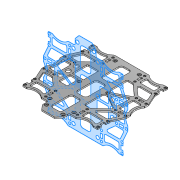
# Autodesk Inventor part: 16_039_BOTTOM_CHASSIS_R1
Saved by Autodesk Inventor 2021.2 (Build 252289000, 289)
## iProperties
Created: 2018-08-08
Part Number: 16_039_BOTTOM_CHASSIS_R1
Material: アルミニウム 6061
Document SubType Name: Modeling
Designer: student
Density: 2.7 g/cm^3
Appearance: 機械加工 - アルミニウム
Mass: 38.4013 g
Surface Area: 190.865 cm^2
Volume: 14.2227 cm^3
Author: student
Autodesk Inventor part; units mm, degrees
ref_plane "YZ Plane" through (0, 0, 0) normal (1, 0, 0) x (0, 1, 0)
ref_plane "XZ Plane" through (0, 0, 0) normal (0, 1, 0) x (-1, 0, 0)
ref_plane "XY Plane" through (0, 0, 0) normal (0, 0, 1) x (1, 0, 0)
sketch "スケッチ1" plane through (0, 0, 0) normal (0, 0, 1) x (1, 0, 0)
  arc A0 (80, 0) -> (40, 69.282) centre (0, 0) ccw construction
  line L0 (0, 0) -> (40, 69.282) construction
  line L1 (0, 0) -> (47.25, 0) construction
  circle A1 centre (24.25, 51.532) radius 1.05
  circle A2 centre (24.25, 36.532) radius 1.05
  circle A3 centre (55.75, 51.532) radius 1.05
  circle A4 centre (55.75, 36.532) radius 1.05
  line L2 (57.25, 54.032) -> (51.25, 54.032)
  line L3 (57.25, 54.032) -> (57.25, 52.8549)
  line L4 (57.25, 47.082) -> (55.2607, 47.082)
  line L5 (54.2, 47.082) -> (54.2, 46.0214) construction
  line L6 (54.2, 40.982) -> (55.2607, 40.982) construction
  line L7 (57.25, 40.982) -> (57.25, 37.8549)
  arc A5 (55.2607, 47.082) -> (54.2, 46.0214) centre (54.7303, 46.5517) ccw
  arc A6 (54.2, 42.0427) -> (55.2607, 40.982) centre (54.7303, 41.5124) ccw
  line L8 (55.2607, 47.082) -> (54.2, 47.082) construction
  line L9 (54.2, 46.0214) -> (54.2, 42.0427)
  line L10 (54.2, 42.0427) -> (54.2, 40.982) construction
  line L11 (55.2607, 40.982) -> (57.25, 40.982)
  line L12 (57.25, 34.032) -> (64.75, 17.25)
  line L13 (64.75, 17.25) -> (64.75, 11.25)
  arc A7 (27.0293, 55.7226) -> (50.6808, 53.8542) centre (40, 69.282) ccw
  arc A8 (64.5722, 10.6808) -> (64.5722, -10.6808) centre (80, 0) ccw
  arc A9 (51.25, 54.032) -> (50.6808, 53.8542) centre (51.25, 53.032) ccw
  arc A10 (27.0293, 55.7226) -> (26.3381, 56) centre (26.3381, 55) ccw
  line L14 (22.7, 40.982) -> (23.7607, 40.982) construction
  line L15 (25.8, 40.982) -> (25.8, 42.0427) construction
  line L16 (25.8, 47.082) -> (24.7393, 47.082) construction
  line L17 (22.7, 47.082) -> (22.7, 46.0214) construction
  arc A11 (22.7, 42.0427) -> (23.7607, 40.982) centre (23.2303, 41.5124) ccw
  arc A12 (23.7607, 47.082) -> (22.7, 46.0214) centre (23.2303, 46.5517) ccw
  arc A13 (25.8, 46.0214) -> (24.7393, 47.082) centre (25.2697, 46.5517) ccw
  arc A14 (24.7393, 40.982) -> (25.8, 42.0427) centre (25.2697, 41.5124) ccw
  line L18 (22.7, 46.0214) -> (22.7, 42.0427)
  line L19 (23.7607, 47.082) -> (22.7, 47.082) construction
  line L20 (24.7393, 47.082) -> (23.7607, 47.082)
  line L21 (25.8, 46.0214) -> (25.8, 47.082) construction
  line L22 (24.7393, 40.982) -> (25.8, 40.982) construction
  line L23 (25.8, 42.0427) -> (25.8, 46.0214)
  line L24 (23.7607, 40.982) -> (24.7393, 40.982)
  line L25 (22.7, 42.0427) -> (22.7, 40.982) construction
  line L26 (0, 56) -> (0, 0)
  arc A15 (64.5722, 10.6808) -> (64.75, 11.25) centre (63.75, 11.25) ccw
  line L27 (57.8, 17.3) -> (56.7393, 17.3) construction
  line L28 (51.7, 17.3) -> (51.7, 16.2393) construction
  line L29 (51.7, 14.2) -> (52.7607, 14.2) construction
  line L30 (57.8, 14.2) -> (57.8, 15.2607) construction
  arc A16 (52.7607, 17.3) -> (51.7, 16.2393) centre (52.2303, 16.7697) ccw
  arc A17 (51.7, 15.2607) -> (52.7607, 14.2) centre (52.2303, 14.7303) ccw
  arc A18 (56.7393, 14.2) -> (57.8, 15.2607) centre (57.2697, 14.7303) ccw
  arc A19 (57.8, 16.2393) -> (56.7393, 17.3) centre (57.2697, 16.7697) ccw
  line L31 (57.8, 16.2393) -> (57.8, 17.3) construction
  line L32 (56.7393, 17.3) -> (52.7607, 17.3)
  line L33 (57.8, 15.2607) -> (57.8, 16.2393)
  line L34 (56.7393, 14.2) -> (57.8, 14.2) construction
  line L35 (52.7607, 14.2) -> (56.7393, 14.2)
  line L36 (51.7, 15.2607) -> (51.7, 14.2) construction
  line L37 (51.7, 16.2393) -> (51.7, 15.2607)
  line L38 (52.7607, 17.3) -> (51.7, 17.3) construction
  circle A20 centre (62.25, 15.75) radius 1.05
  circle A21 centre (47.25, 15.75) radius 1.05
  line L39 (46.5207, 19.8) -> (56.1447, 19.8)
  line L40 (57.9706, 22.616) -> (53.2861, 33.0981)
  arc A22 (56.1447, 19.8) -> (57.9706, 22.616) centre (56.1447, 21.8) ccw
  arc A23 (31.5743, 49.2149) -> (48.4257, 49.2149) centre (40, 69.282) ccw
  line L41 (28.8, 47.3709) -> (28.8, 40.782)
  line L42 (30.8, 38.782) -> (49.2, 38.782)
  line L43 (51.2, 40.782) -> (51.2, 47.3709)
  arc A24 (31.5743, 49.2149) -> (28.8, 47.3709) centre (30.8, 47.3709) ccw
  arc A25 (51.2, 47.3709) -> (48.4257, 49.2149) centre (49.2, 47.3709) ccw
  arc A26 (49.2, 38.782) -> (51.2, 40.782) centre (49.2, 40.782) ccw
  arc A27 (28.8, 40.782) -> (30.8, 38.782) centre (30.8, 40.782) ccw
  line L44 (24.25, 36.532) -> (47.25, 15.75) construction
  line L45 (34.9199, 34.282) -> (51.4602, 34.282)
  line L46 (45.1798, 20.316) -> (33.5791, 30.7981)
  line L47 (54.3774, 36.532) -> (35.8774, 36.532) construction
  arc A28 (34.9199, 34.282) -> (33.5791, 30.7981) centre (34.9199, 32.282) ccw
  circle A29 centre (47.25, -15.75) radius 1.05 construction
  line L48 (47.25, -9.2) -> (47.25, 9.2)
  line L49 (49.25, 11.2) -> (58.0888, 11.2)
  arc A30 (59.9329, 8.4257) -> (59.9329, -8.4257) centre (80, 0) ccw
  arc A31 (49.25, 11.2) -> (47.25, 9.2) centre (49.25, 9.2) ccw
  arc A32 (59.9329, 8.4257) -> (58.0888, 11.2) centre (58.0888, 9.2) ccw
  line L50 (47.25, 0) -> (58.2358, 0) construction
  line L51 (58.2358, 0) -> (80, 0) construction
  line L52 (47.25, 0) -> (58.2358, 0) construction
  arc A33 (53.2861, 33.0981) -> (51.4602, 34.282) centre (51.4602, 32.282) ccw
  arc A34 (45.1798, 20.316) -> (46.5207, 19.8) centre (46.5207, 21.8) ccw
  line L53 (47.25, 15.75) -> (47.25, 0) construction
  line L54 (26.3381, 56) -> (0, 56)
  circle A35 centre (24.25, -51.532) radius 1.05
  circle A36 centre (24.25, -36.532) radius 1.05
  circle A37 centre (55.75, -36.532) radius 1.05
  line L55 (57.25, -54.032) -> (51.25, -54.032)
  line L56 (57.25, -47.082) -> (55.2607, -47.082)
  arc A38 (54.2, -46.0214) -> (55.2607, -47.082) centre (54.7303, -46.5517) ccw
  arc A39 (55.2607, -40.982) -> (54.2, -42.0427) centre (54.7303, -41.5124) ccw
  line L57 (54.2, -46.0214) -> (54.2, -42.0427)
  line L58 (55.2607, -40.982) -> (57.25, -40.982)
  arc A40 (50.6808, -53.8542) -> (27.0293, -55.7226) centre (40, -69.282) ccw
  arc A41 (50.6808, -53.8542) -> (51.25, -54.032) centre (51.25, -53.032) ccw
  arc A42 (26.3381, -56) -> (27.0293, -55.7226) centre (26.3381, -55) ccw
  line L59 (22.7, -40.982) -> (23.7607, -40.982) construction
  line L60 (25.8, -40.982) -> (25.8, -42.0427) construction
  line L61 (25.8, -47.082) -> (24.7393, -47.082) construction
  line L62 (22.7, -47.082) -> (22.7, -46.0214) construction
  arc A43 (23.7607, -40.982) -> (22.7, -42.0427) centre (23.2303, -41.5124) ccw
  arc A44 (22.7, -46.0214) -> (23.7607, -47.082) centre (23.2303, -46.5517) ccw
  arc A45 (24.7393, -47.082) -> (25.8, -46.0214) centre (25.2697, -46.5517) ccw
  arc A46 (25.8, -42.0427) -> (24.7393, -40.982) centre (25.2697, -41.5124) ccw
  line L63 (22.7, -46.0214) -> (22.7, -42.0427)
  line L64 (23.7607, -47.082) -> (22.7, -47.082) construction
  line L65 (24.7393, -47.082) -> (23.7607, -47.082)
  line L66 (25.8, -46.0214) -> (25.8, -47.082) construction
  line L67 (24.7393, -40.982) -> (25.8, -40.982) construction
  line L68 (25.8, -42.0427) -> (25.8, -46.0214)
  line L69 (23.7607, -40.982) -> (24.7393, -40.982)
  line L70 (22.7, -42.0427) -> (22.7, -40.982) construction
  arc A47 (64.75, -11.25) -> (64.5722, -10.6808) centre (63.75, -11.25) ccw
  line L71 (57.8, -17.3) -> (56.7393, -17.3) construction
  line L72 (51.7, -17.3) -> (51.7, -16.2393) construction
  line L73 (51.7, -14.2) -> (52.7607, -14.2) construction
  line L74 (57.8, -14.2) -> (57.8, -15.2607) construction
  arc A48 (51.7, -16.2393) -> (52.7607, -17.3) centre (52.2303, -16.7697) ccw
  arc A49 (52.7607, -14.2) -> (51.7, -15.2607) centre (52.2303, -14.7303) ccw
  arc A50 (57.8, -15.2607) -> (56.7393, -14.2) centre (57.2697, -14.7303) ccw
  arc A51 (56.7393, -17.3) -> (57.8, -16.2393) centre (57.2697, -16.7697) ccw
  line L75 (57.8, -16.2393) -> (57.8, -17.3) construction
  line L76 (56.7393, -17.3) -> (52.7607, -17.3)
  line L77 (57.8, -15.2607) -> (57.8, -16.2393)
  line L78 (56.7393, -14.2) -> (57.8, -14.2) construction
  line L79 (52.7607, -14.2) -> (56.7393, -14.2)
  line L80 (51.7, -15.2607) -> (51.7, -14.2) construction
  line L81 (51.7, -16.2393) -> (51.7, -15.2607)
  line L82 (52.7607, -17.3) -> (51.7, -17.3) construction
  circle A52 centre (62.25, -15.75) radius 1.05
  circle A53 centre (47.25, -15.75) radius 1.05
  line L83 (46.5207, -19.8) -> (56.1447, -19.8)
  line L84 (57.9706, -22.616) -> (53.2861, -33.0981)
  arc A54 (57.9706, -22.616) -> (56.1447, -19.8) centre (56.1447, -21.8) ccw
  arc A55 (48.4257, -49.2149) -> (31.5743, -49.2149) centre (40, -69.282) ccw
  line L85 (28.8, -47.3709) -> (28.8, -40.782)
  line L86 (30.8, -38.782) -> (49.2, -38.782)
  line L87 (51.2, -40.782) -> (51.2, -47.3709)
  arc A56 (28.8, -47.3709) -> (31.5743, -49.2149) centre (30.8, -47.3709) ccw
  arc A57 (48.4257, -49.2149) -> (51.2, -47.3709) centre (49.2, -47.3709) ccw
  arc A58 (51.2, -40.782) -> (49.2, -38.782) centre (49.2, -40.782) ccw
  arc A59 (30.8, -38.782) -> (28.8, -40.782) centre (30.8, -40.782) ccw
  line L88 (34.9199, -34.282) -> (51.4602, -34.282)
  line L89 (45.1798, -20.316) -> (33.5791, -30.7981)
  arc A60 (33.5791, -30.7981) -> (34.9199, -34.282) centre (34.9199, -32.282) ccw
  line L90 (49.25, -11.2) -> (58.0888, -11.2)
  arc A61 (47.25, -9.2) -> (49.25, -11.2) centre (49.25, -9.2) ccw
  arc A62 (58.0888, -11.2) -> (59.9329, -8.4257) centre (58.0888, -9.2) ccw
  arc A63 (51.4602, -34.282) -> (53.2861, -33.0981) centre (51.4602, -32.282) ccw
  arc A64 (46.5207, -19.8) -> (45.1798, -20.316) centre (46.5207, -21.8) ccw
  line L91 (26.3381, -56) -> (18, -56)
  circle A65 centre (18.5, -51) radius 1.3
  line L92 (0, -72) -> (10, -72)
  line L93 (10, -72) -> (16, -65)
  line L94 (16, -65) -> (16, -58)
  arc A66 (18, -56) -> (16, -58) centre (18, -58) ccw
  line L95 (0, -72) -> (0, 0)
  circle A67 centre (55.75, -51.532) radius 1.05
  circle A68 centre (12.5, -62) radius 1.3
  arc A69 (57.25, 50.2092) -> (57.25, 52.8549) centre (55.75, 51.532) ccw
  line L96 (57.25, 52.8549) -> (57.25, 50.2092) construction
  line L97 (57.25, 50.2092) -> (57.25, 47.082)
  arc A70 (57.25, 35.2092) -> (57.25, 37.8549) centre (55.75, 36.532) ccw
  line L98 (57.25, 37.8549) -> (57.25, 35.2092) construction
  line L99 (57.25, 35.2092) -> (57.25, 34.032)
  arc A71 (57.25, -52.8549) -> (57.25, -50.2092) centre (55.75, -51.532) ccw
  arc A72 (57.25, -37.8549) -> (57.25, -35.2092) centre (55.75, -36.532) ccw
  line L100 (57.25, -40.982) -> (57.25, -37.8549)
  line L101 (57.25, -35.2092) -> (57.25, -34.032)
  line L102 (57.25, -54.032) -> (57.25, -52.8549)
  line L103 (57.25, -50.2092) -> (57.25, -47.082)
  line L104 (57.25, -34.032) -> (64.75, -17.25)
  line L105 (64.75, -17.25) -> (64.75, -11.25)
  circle A73 centre (18.5, 49) radius 1.3
  line L106 (24.25, 36.532) -> (55.75, 36.532) construction
  line L107 (55.75, 36.532) -> (55.75, 51.532) construction
  line L108 (55.75, 51.532) -> (24.25, 51.532) construction
  line L109 (24.25, 51.532) -> (24.25, 36.532) construction
  line L110 (47.25, -15.75) -> (62.25, -15.75) construction
  line L111 (62.25, -15.75) -> (62.25, 15.75) construction
  line L112 (62.25, 15.75) -> (47.25, 15.75) construction
  line L113 (47.25, 15.75) -> (47.25, -15.75) construction
  line L114 (24.25, -51.532) -> (55.75, -51.532) construction
  line L115 (55.75, -51.532) -> (55.75, -36.532) construction
  line L116 (55.75, -36.532) -> (24.25, -36.532) construction
  line L117 (24.25, -36.532) -> (24.25, -51.532) construction
  line L118 (40, 69.282) -> (40, 30.0989) construction
  line L119 (17.2482, 44.032) -> (63.5437, 44.032) construction
  line L120 (54.75, 18.203) -> (54.75, -19.0893) construction
  point P0 (50.9332, 54.032)
  point P1 (64.75, 10.9332)
  point P2 (55.2496, 28.7046)
  point P3 (28.8, 50.6208)
  point P4 (51.2, 50.6208)
  point P5 (61.3388, 11.2)
  point P6 (45.25, 13.125)
  point P7 (55.2496, -28.7046)
  dimension "d3" = 60
  dimension "d7" = 2.1
  dimension "d10" = 3.05
  dimension "d11" = 0.75
  dimension "d13" = 1
  dimension "d14" = 1
  dimension "d15" = 6
  dimension "d20" = 0.75
  dimension "d21" = 1
  dimension "d22" = 6
  dimension "d27" = 0.75
  dimension "d28" = 2.1
  dimension "d29" = 6.95
  dimension "d31" = 4
  dimension "d32" = 2.5
  dimension "d34" = 3
  dimension "d35" = 3
  dimension "d36" = 3
  dimension "d38" = 2
  dimension "d40" = 4.5
  dimension "d41" = 2
  dimension "d42" = 4
  dimension "d48" = 2
  dimension "d49" = 3
  dimension "d50" = 3
  dimension "d54" = 2
  dimension "d55" = 2
  dimension "d67" = 56
  dimension "d78" = 80
  dimension "d80" = 2
  dimension "d81" = 72
  dimension "d82" = 16
  dimension "d83" = 6
  dimension "d84" = 7
  dimension "d113" = 2
  dimension "d119" = 2.6
  dimension "d132" = 48.5
  dimension "d133" = 31.5
  dimension "d134" = 15
  dimension "d135" = 15
  dimension "d136" = 15
  dimension "d137" = 31.5
  dimension "d138" = 31.5
  dimension "d139" = 49
  dimension "d140" = 37
  dimension "d141" = 25
  dimension "d142" = 62
  dimension "d143" = 37
  dimension "d144" = 51
  dimension "d145" = 17.75
  dimension "d146" = 17.75
  dimension "d147" = 22.4
  dimension "d148" = 22.4
  dimension "d149" = 2.25
  dimension "d150" = 2.5
  dimension "d151" = 18.7642
  dimension "d152" = 3.1
  dimension "d153" = 6.1
  dimension "d154" = 6.1
  dimension "d155" = 25.25
  dimension "d156" = 25.25
  dimension "d157" = 6.1
  constraints: 243 end point, 132 point on circle, 96 symmetric about line, 74 centre point, 44 parallel, 42 perpendicular, 28 tangent, 20 equal radius, 20 horizontal, 12 point on line, 10 collinear, 8 vertical, 5 coincident, 4 concentric, 1 midpoint, 39 other
  measures "d3" angle of L1 L0
  measures "d7" diameter of A4
  measures "d10" distance between parallel lines of L5 L3
  measures "d11" radius of A5
  measures "d13" radius of A9
  measures "d14" radius of A10
  measures "d15" distance of L2.start L2.end
  measures "d20" radius of A11
  measures "d21" radius of A15
  measures "d22" distance of L12.end L13.end
  measures "d27" radius of A16
  measures "d28" diameter of A20
  measures "d29" distance of L7.start L12.start
  measures "d31" distance between parallel lines of L12 L40
  measures "d32" distance between parallel lines of L32 L39
  measures "d34" radial gap between concentric circles of A23 A7
  measures "d35" distance between parallel lines of L9 L43
  measures "d36" distance between parallel lines of L41 L23
  measures "d38" radius of A24
  measures "d40" distance between parallel lines of L45 L42
  measures "d41" radius of A28
  measures "d42" diameter of L46 L44
  measures "d48" radius of A31
  measures "d49" radial gap between concentric circles of A8 A30
  measures "d50" distance between parallel lines of L35 L49
  measures "d54" radius of A33
  measures "d55" radius of A22
  measures "d67" distance of L26.start L0.start
  measures "d78" radius of A0
  measures "d80" radius of A66
  measures "d81" distance of L92.start L0.start
  measures "d82" distance between parallel lines of L95 L94
  measures "d83" distance from line of L94 L92.end
  measures "d84" distance from line of L92 L93.end
  measures "d113" radius of A69
  measures "d119" diameter of A65
  measures "d132" diameter of L109 L26
  measures "d133" distance between parallel lines of L107 L109
  measures "d134" distance between parallel lines of L108 L106
  measures "d135" distance between parallel lines of L116 L114
  measures "d136" distance between parallel lines of L111 L113
  measures "d137" distance between parallel lines of L115 L117
  measures "d138" distance between parallel lines of L112 L110
  measures "d139" distance from line of A73.centre L1
  measures "d140" diameter of A73.centre L26
  measures "d141" diameter of A68.centre L95
  measures "d142" distance from line of L1 A68.centre
  measures "d143" diameter of A65.centre L95
  measures "d144" distance from line of L1 A65.centre
  measures "d145" distance from line of A40.centre L114
  measures "d146" distance from line of L111 L51.end
  measures "d147" distance between parallel lines of L41 L43
  measures "d148" distance between parallel lines of L90 L49
  measures "d149" distance between parallel lines of L86 L116
  measures "d150" distance between parallel lines of L13 L111
  measures "d151" radius of A8
  measures "d152" distance between parallel lines of L23 L18
  measures "d153" distance between parallel lines of L24 L20
  measures "d154" distance between parallel lines of L11 L4
  measures "d155" distance from line of L119 L0.end
  measures "d156" distance from line of L51.end L120
  measures "d157" distance between parallel lines of L77 L81
extrude "押し出し1" add sketch "スケッチ1" along normal blind 2
chamfer "面取り1" distance 0.5 angle 45 1 edges at (57.25, -54.032, 1)
chamfer "面取り2" distance 0.25 angle 45 4 edges at (57.25, -40.982, 1) (57.25, -47.082, 1) (57.25, 40.982, 1) (57.25, 47.082, 1)
mirror "ミラー2" about plane through (0, 0, 0) normal (1, 0, 0) of "押し出し1", "面取り1", "面取り2"
sketch "スケッチ3" plane through (0, 0, 2) normal (0, 0, 1) x (1, 0, 0)
  circle A0 centre (-41.3, -12) radius 3.45
  circle A1 centre (-41.3, 0) radius 3.45
  circle A2 centre (-41.3, 12) radius 3.45
  line L0 (-37.85, -22) -> (-37.85, 22) construction
  line L1 (-44.75, 12.25) -> (-44.75, -12.25) construction
  circle A3 centre (47.25, 15.75) radius 1.05 construction
  arc A4 (16, 8.7246) -> (22.5141, 4.7453) centre (20.4725, 8.7246) ccw
  line L2 (22.5141, 4.7453) -> (41.5805, 14.5272)
  line L3 (42.0084, 17.7906) -> (25.7115, 32.516)
  line L4 (24.3706, 33.032) -> (18, 33.032)
  line L5 (16, 31.032) -> (16, 8.7246)
  arc A5 (18, 33.032) -> (16, 31.032) centre (18, 31.032) ccw
  arc A6 (25.7115, 32.516) -> (24.3706, 33.032) centre (24.3706, 31.032) ccw
  arc A7 (41.5805, 14.5272) -> (42.0084, 17.7906) centre (40.6676, 16.3067) ccw
  line L6 (45.1798, 20.316) -> (33.5791, 30.7981) construction
  line L7 (34.9199, 34.282) -> (51.4602, 34.282) construction
  circle A8 centre (18.5, 1) radius 1.4
  line L8 (-4, 48) -> (4, 48)
  line L9 (8, 44) -> (8, 19.6667)
  line L10 (4, 15.6667) -> (-4, 15.6667)
  line L11 (-8, 19.6667) -> (-8, 44)
  line L12 (-4, 9.6667) -> (4, 9.6667)
  line L13 (8, 5.6667) -> (8, -18.6667)
  line L14 (4, -22.6667) -> (-4, -22.6667)
  line L15 (-8, -18.6667) -> (-8, 5.6667)
  line L16 (-4, -28.6667) -> (4, -28.6667)
  line L17 (8, -32.6667) -> (8, -57)
  line L18 (4, -61) -> (-4, -61)
  line L19 (-8, -57) -> (-8, -32.6667)
  arc A9 (-4, -28.6667) -> (-8, -32.6667) centre (-4, -32.6667) ccw
  arc A10 (8, -32.6667) -> (4, -28.6667) centre (4, -32.6667) ccw
  arc A11 (4, -61) -> (8, -57) centre (4, -57) ccw
  arc A12 (-8, -57) -> (-4, -61) centre (-4, -57) ccw
  arc A13 (-8, -18.6667) -> (-4, -22.6667) centre (-4, -18.6667) ccw
  arc A14 (4, -22.6667) -> (8, -18.6667) centre (4, -18.6667) ccw
  arc A15 (8, 5.6667) -> (4, 9.6667) centre (4, 5.6667) ccw
  arc A16 (-4, 9.6667) -> (-8, 5.6667) centre (-4, 5.6667) ccw
  arc A17 (-8, 19.6667) -> (-4, 15.6667) centre (-4, 19.6667) ccw
  arc A18 (4, 15.6667) -> (8, 19.6667) centre (4, 19.6667) ccw
  arc A19 (8, 44) -> (4, 48) centre (4, 44) ccw
  arc A20 (-4, 48) -> (-8, 44) centre (-4, 44) ccw
  line L20 (0, 0) -> (0, 60.956) construction
  line L21 (26.3381, 56) -> (-26.3381, 56) construction
  line L22 (7, -66) -> (-7, -66) construction
  circle A21 centre (-18.5, -5.95) radius 1.4
  line L23 (40.3371, 10.5175) -> (24.8744, 2.5845)
  line L24 (24.7806, -0.9231) -> (40.2432, -9.9318)
  line L25 (43.25, -8.2037) -> (43.25, 8.738)
  arc A22 (43.25, 8.738) -> (40.3371, 10.5175) centre (41.25, 8.738) ccw
  arc A23 (40.2432, -9.9318) -> (43.25, -8.2037) centre (41.25, -8.2037) ccw
  arc A24 (24.8744, 2.5845) -> (24.7806, -0.9231) centre (25.7874, 0.805) ccw
  line L26 (47.25, -9.2) -> (47.25, 9.2) construction
  arc A25 (22.1904, -2.8861) -> (16, -6.4438) centre (20.1176, -6.4438) ccw
  line L27 (22.1904, -2.8861) -> (41.9038, -14.3713)
  line L28 (42.2378, -17.5833) -> (25.7115, -32.516)
  line L29 (24.3706, -33.032) -> (18, -33.032)
  line L30 (16, -31.032) -> (16, -6.4438)
  arc A26 (16, -31.032) -> (18, -33.032) centre (18, -31.032) ccw
  arc A27 (24.3706, -33.032) -> (25.7115, -32.516) centre (24.3706, -31.032) ccw
  arc A28 (42.2378, -17.5833) -> (41.9038, -14.3713) centre (40.897, -16.0994) ccw
  arc A29 (19.5294, -2.3452) -> (19.5294, 4.3452) centre (18.5, 1) ccw construction
  line L31 (0, 0) -> (14.0478, 0) construction
  line L32 (47.25, 15.75) -> (18.5, 1) construction
  circle A30 centre (47.25, -15.75) radius 1.05 construction
  line L33 (18.5, 1) -> (47.25, -15.75) construction
  line L34 (33.5791, -30.7981) -> (45.1798, -20.316) construction
  line L35 (-41.3, 12) -> (-41.3, 0) construction
  line L36 (-41.3, 0) -> (-41.3, -12) construction
  line L37 (-41.3, 0) -> (0, 0) construction
  circle A31 centre (24.25, 36.532) radius 1.05 construction
  circle A32 centre (55.75, 36.532) radius 1.05 construction
  line L38 (24.25, 36.532) -> (55.75, 36.532) construction
  line L39 (-18.55, 0.55) -> (-33.85, 0.55) construction
  line L40 (-18.55, 22) -> (-18.55, 0.55) construction
  line L41 (-33.85, 22) -> (-18.55, 22) construction
  line L42 (-33.85, 0.55) -> (-33.85, 22) construction
  line L43 (-33.85, -20) -> (-33.85, -4.65) construction
  line L44 (-23, -20) -> (-33.85, -20) construction
  line L45 (-23, -4.65) -> (-23, -20) construction
  line L46 (-33.85, -4.65) -> (-23, -4.65) construction
  line L47 (-34.85, -20) -> (-34.85, -4.65)
  line L48 (-33.85, -3.65) -> (-23, -3.65)
  line L49 (-22, -4.65) -> (-22, -20)
  line L50 (-23, -21) -> (-33.85, -21)
  arc A33 (-33.85, -3.65) -> (-34.85, -4.65) centre (-33.85, -4.65) ccw
  arc A34 (-22, -4.65) -> (-23, -3.65) centre (-23, -4.65) ccw
  arc A35 (-23, -21) -> (-22, -20) centre (-23, -20) ccw
  arc A36 (-34.85, -20) -> (-33.85, -21) centre (-33.85, -20) ccw
  line L51 (-33.85, -0.45) -> (-18.55, -0.45)
  line L52 (-17.55, 0.55) -> (-17.55, 22)
  line L53 (-18.55, 23) -> (-33.85, 23)
  line L54 (-34.85, 22) -> (-34.85, 0.55)
  arc A37 (-18.55, -0.45) -> (-17.55, 0.55) centre (-18.55, 0.55) ccw
  arc A38 (-34.85, 0.55) -> (-33.85, -0.45) centre (-33.85, 0.55) ccw
  arc A39 (-33.85, 23) -> (-34.85, 22) centre (-33.85, 22) ccw
  arc A40 (-17.55, 22) -> (-18.55, 23) centre (-18.55, 22) ccw
  point P0 (-8, 9.6667)
  point P1 (8, -22.6667)
  point P2 (-8, -28.6667)
  point P3 (8, -61)
  point P4 (34.9199, -34.282)
  dimension "d89" = 2
  dimension "d90" = 4
  dimension "d95" = 2.8
  dimension "d97" = 8
  dimension "d98" = 5
  dimension "d99" = 6
  dimension "d100" = 6
  dimension "d101" = 16
  dimension "d115" = 2
  dimension "d117" = 4
  dimension "d120" = 2
  dimension "d121" = 3
  dimension "d122" = 3
  dimension "d123" = 32
  dimension "d124" = 4
  dimension "d125" = 4
  dimension "d126" = 12
  dimension "d127" = 3.5
  dimension "d128" = 1
  dimension "d129" = 1
  dimension "d130" = 1
  dimension "d131" = 1
  dimension "d158" = 37
  dimension "d159" = 5.95
  constraints: 78 end point, 66 tangent, 62 point on circle, 36 centre point, 26 equal radius, 12 point on line, 10 parallel, 6 horizontal, 4 collinear, 4 perpendicular, 4 vertical, 1 concentric, 10 other
  measures "d89" radius of A5
  measures "d90" distance between parallel lines of L6 L3
  measures "d95" diameter of A8
  measures "d97" distance between parallel lines of L21 L8
  measures "d98" distance between parallel lines of L18 L22
  measures "d99" distance between parallel lines of L12 L10
  measures "d100" distance between parallel lines of L16 L14
  measures "d101" distance between parallel lines of L9 L11
  measures "d115" radius of A24
  measures "d117" distance between parallel lines of L26 L25
  measures "d120" radius of A22
  measures "d121" distance between parallel lines of L23 L2
  measures "d122" distance between parallel lines of L27 L24
  measures "d123" diameter of L5 L20
  measures "d124" distance between parallel lines of L34 L28
  measures "d125" radius of A15
  measures "d126" distance of L35.end L36.end
  measures "d127" distance between parallel lines of L4 L38
  measures "d128" distance between parallel lines of L44 L50
  measures "d129" radius of A33
  measures "d130" distance between parallel lines of L39 L51
  measures "d131" radius of A37
  measures "d158" diameter of A21.centre L20
  measures "d159" distance from line of L37 A21.centre
extrude "押し出し3" cut sketch "スケッチ3" against normal blind 2
sketch "スケッチ4" plane through (0, 0, 2) normal (0, 0, 1) x (1, 0, 0)
  line L0 (0, 0) -> (0, -67.8124) construction
  circle A0 centre (55.75, 51.532) radius 1.05 projected
  circle A1 centre (55.75, 51.532) radius 1.7
  circle A2 centre (55.75, 36.532) radius 1.05 projected
  circle A3 centre (55.75, 36.532) radius 1.7
  circle A4 centre (24.25, 36.532) radius 1.05 projected
  circle A5 centre (24.25, 36.532) radius 1.7
  circle A6 centre (24.25, 51.532) radius 1.05 projected
  circle A7 centre (24.25, 51.532) radius 1.7
  circle A8 centre (62.25, 15.75) radius 1.05 projected
  circle A9 centre (62.25, 15.75) radius 1.7
  circle A10 centre (47.25, 15.75) radius 1.05 projected
  circle A11 centre (47.25, 15.75) radius 1.7
  circle A12 centre (47.25, -15.75) radius 1.05 projected
  circle A13 centre (47.25, -15.75) radius 1.7
  circle A14 centre (62.25, -15.75) radius 1.05 projected
  circle A15 centre (62.25, -15.75) radius 1.7
  line L1 (0, 0) -> (12.4062, 0) construction
  circle A16 centre (55.75, -51.532) radius 1.05
  circle A17 centre (55.75, -51.532) radius 1.7
  circle A18 centre (55.75, -36.532) radius 1.05
  circle A19 centre (55.75, -36.532) radius 1.7
  circle A20 centre (24.25, -36.532) radius 1.05
  circle A21 centre (24.25, -36.532) radius 1.7
  circle A22 centre (24.25, -51.532) radius 1.05
  circle A23 centre (24.25, -51.532) radius 1.7
  circle A24 centre (18.5, 1) radius 2.6
  circle A25 centre (18.5, -51) radius 1.3 projected
  circle A26 centre (18.5, -51) radius 2.6
  circle A27 centre (12.5, -62) radius 1.3 projected
  circle A28 centre (12.5, -62) radius 2.6
  circle A29 centre (-18.5, -51) radius 1.3
  circle A30 centre (-18.5, -51) radius 2.6
  circle A31 centre (-12.5, -62) radius 1.3
  circle A32 centre (-12.5, -62) radius 2.6
  circle A33 centre (-55.75, 51.532) radius 1.05
  circle A34 centre (-55.75, 51.532) radius 1.7
  circle A35 centre (-55.75, 36.532) radius 1.05
  circle A36 centre (-55.75, 36.532) radius 1.7
  circle A37 centre (-24.25, 36.532) radius 1.05
  circle A38 centre (-24.25, 36.532) radius 1.7
  circle A39 centre (-24.25, 51.532) radius 1.05
  circle A40 centre (-24.25, 51.532) radius 1.7
  circle A41 centre (-62.25, 15.75) radius 1.05
  circle A42 centre (-62.25, 15.75) radius 1.7
  circle A43 centre (-47.25, 15.75) radius 1.05
  circle A44 centre (-47.25, 15.75) radius 1.7
  circle A45 centre (-47.25, -15.75) radius 1.05
  circle A46 centre (-47.25, -15.75) radius 1.7
  circle A47 centre (-62.25, -15.75) radius 1.05
  circle A48 centre (-62.25, -15.75) radius 1.7
  circle A49 centre (-55.75, -36.532) radius 1.05
  circle A50 centre (-55.75, -36.532) radius 1.7
  circle A51 centre (-55.75, -51.532) radius 1.05
  circle A52 centre (-55.75, -51.532) radius 1.7
  circle A53 centre (-24.25, -36.532) radius 1.05
  circle A54 centre (-24.25, -36.532) radius 1.7
  circle A55 centre (-24.25, -51.532) radius 1.05
  circle A56 centre (-24.25, -51.532) radius 1.7
  circle A57 centre (-18.5, -5.95) radius 2.6
  circle A58 centre (18.5, 49) radius 1.3 projected
  circle A59 centre (-18.5, 49) radius 1.3 projected
  circle A60 centre (18.5, 49) radius 2.6
  circle A61 centre (-18.5, 49) radius 2.6
  circle A62 centre (18.5, 1) radius 1.4 projected
  circle A63 centre (-18.5, -5.95) radius 1.4 projected
  dimension "d109" = 3.4
  dimension "d110" = 5.2
  constraints: 50 centre point, 36 symmetric about line, 32 coincident, 12 equal radius, 4 end point, 2 concentric, 1 horizontal, 1 vertical, 36 other
  measures "d109" diameter of A3
  measures "d110" diameter of A24
extrude "押し出し4" cut sketch "スケッチ4" against normal blind 0.8 contours A0 | A1 | A2 | A3 | A4 | A5 | A6 | A7 | A8 | A9 | A10 | A11 | A12 | A13 | A14 | A15 | A16 | A17 | A18 | A19 | A20 | A21 | A22 | A23 | A24 | A25 | A26 | A27 | A28 | A29 | A30 | A31 | A32 | A33 | A34 | A35 | A36 | A37 | A38 | A39 | A40 | A41 | A42 | A43 | A44 | A45 | A46 | A47 | A48 | A49 | A50 | A51 | A52 | A53 | A54 | A55 | A56 | A57 | A60 | A61 | A62 | A63
